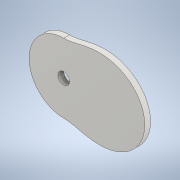
# Autodesk Inventor part: Disc Cam
Saved by Autodesk Inventor 2020.2 (Build 242310000, 310)
## iProperties
Created: 2020-01-12
Part Number: Disc Cam
Material: Stainless Steel, Austenitic
Document SubType Name: Modeling
Designer: robst
Manufacturer: Standard
Standards Organization: Custom
Density: 1 g/cm^3
Appearance: Steel
CustomPartVersion: 1
Author: robst
Autodesk Inventor part; units mm, degrees
ref_plane "YZ Plane" through (0, 0, 0) normal (1, 0, 0) x (0, 1, 0)
ref_plane "XZ Plane" through (0, 0, 0) normal (0, 1, 0) x (-1, 0, 0)
ref_plane "XY Plane" through (0, 0, 0) normal (0, 0, 1) x (1, 0, 0)
sketch "Main Sketch" plane through (0, 0, 0) normal (0, 0, 1) x (1, 0, 0)
  spline S0 degree 5 poles (0, 76.2) (2.4415, 76.2811) (6.8419, 76.4448) (14.3342, 77.0155) (22.5678, 78.9482) (34.573, 81.6506) (46.176, 84.4734) (59.6543, 86.8011) (74.07, 88.0758) (89.5247, 87.6776) (105.5032, 85.1455) (121.5054, 80.094) (136.8136, 72.3306) (150.6942, 61.8554) (162.4064, 48.8865) (171.2981, 33.8414) (176.8529, 17.3087) (178.7423, 0) (176.8529, -17.3087) (171.2981, -33.8414) (162.4064, -48.8865) (150.6941, -61.8554) (136.8137, -72.3305) (121.5052, -80.0941) (105.5037, -85.1453) (89.5236, -87.678) (74.0723, -88.0749) (59.6496, -86.803) (46.1853, -84.4696) (34.1732, -81.5655) (22.4222, -78.8937) (12.4959, -76.6296) (0.313, -76.0937) (-7.0815, -76.2043) (-15.7981, -74.7442) (-23.5043, -72.7115) (-31.1018, -69.794) (-38.1945, -66.1763) (-44.9165, -61.8146) (-51.1259, -56.7839) (-56.7839, -51.1274) (-61.816, -44.9123) (-66.1725, -38.2045) (-69.8032, -31.0785) (-72.6695, -23.6117) (-74.7395, -15.8864) (-75.9906, -7.9869) (-76.4092, 0) (-75.9906, 7.9869) (-74.7395, 15.8864) (-72.6695, 23.6117) (-69.8032, 31.0785) (-66.1725, 38.2045) (-61.8159, 44.9124) (-56.7843, 51.1273) (-51.1251, 56.7841) (-44.9184, 61.8141) (-38.1902, 66.1776) (-31.112, 69.7909) (-23.837, 72.5819) (-16.3649, 74.6032) (-9.6201, 75.7956) (-5.285, 76.037) (-2.0624, 76.1315) (0, 76.2) knots 0 0 0 0 0 0 0.019966 0.033509 0.050708 0.068396 0.086675 0.105572 0.125041 0.144982 0.165276 0.1858 0.206452 0.22715 0.247846 0.26852 0.289177 0.309833 0.330508 0.351204 0.371902 0.392553 0.413078 0.433371 0.453313 0.472781 0.491679 0.509958 0.527646 0.544844 0.561198 0.57685 0.591915 0.606464 0.620518 0.634573 0.648628 0.662683 0.676738 0.690793 0.704848 0.718903 0.732957 0.747012 0.761067 0.775122 0.789177 0.803232 0.817287 0.831342 0.845396 0.859451 0.873506 0.887561 0.901616 0.915671 0.929726 0.943781 0.957835 0.97189 0.983134 1 1 1 1 1 1
  point P0 (22.0134, 78.8258)
  point P1 (33.3701, 81.4116)
  point P2 (45.5354, 84.1258)
  point P3 (58.8273, 86.3979)
  point P4 (73.3136, 87.6269)
  point P5 (88.8039, 87.2207)
  point P6 (104.8783, 84.6627)
  point P7 (120.9362, 79.576)
  point P8 (136.2611, 71.7733)
  point P9 (150.0945, 61.2842)
  point P10 (161.7111, 48.3549)
  point P11 (170.4865, 33.4236)
  point P12 (175.947, 17.0772)
  point P13 (177.8, 0)
  point P14 (175.947, -17.0772)
  point P15 (170.4865, -33.4236)
  point P16 (161.7111, -48.3549)
  point P17 (150.0945, -61.2842)
  point P18 (136.2611, -71.7733)
  point P19 (120.9362, -79.576)
  point P20 (104.8783, -84.6627)
  point P21 (88.8039, -87.2207)
  point P22 (73.3136, -87.6269)
  point P23 (58.8273, -86.3979)
  point P24 (45.5354, -84.1258)
  point P25 (33.3701, -81.4116)
  point P26 (22.0134, -78.8258)
  point P27 (11.002, -76.9174)
  point P28 (0, -76.2)
  point P29 (-7.9651, -75.7826)
  point P30 (-15.8429, -74.5348)
  point P31 (-23.5471, -72.4705)
  point P32 (-30.9933, -69.6122)
  point P33 (-38.1, -65.9911)
  point P34 (-44.7892, -61.6471)
  point P35 (-50.9878, -56.6276)
  point P36 (-56.6276, -50.9878)
  point P37 (-61.6471, -44.7892)
  point P38 (-65.9911, -38.1)
  point P39 (-69.6122, -30.9933)
  point P40 (-72.4705, -23.5471)
  point P41 (-74.5348, -15.8429)
  point P42 (-75.7826, -7.9651)
  point P43 (-76.2, 0)
  point P44 (-75.7826, 7.9651)
  point P45 (-74.5348, 15.8429)
  point P46 (-72.4705, 23.5471)
  point P47 (-69.6122, 30.9933)
  point P48 (-65.9911, 38.1)
  point P49 (-61.6471, 44.7892)
  point P50 (-56.6276, 50.9878)
  point P51 (-50.9878, 56.6276)
  point P52 (-44.7892, 61.6471)
  point P53 (-38.1, 65.9911)
  point P54 (-30.9933, 69.6122)
  point P55 (-23.5471, 72.4705)
  point P56 (-15.8429, 74.5348)
  point P57 (-7.9651, 75.7826)
  constraints: 60 other
extrude "Cam" add sketch "Main Sketch" along normal blind 12.7
sketch "Sketch2" plane through (0, 0, 12.7) normal (0, 0, 1) x (1, 0, 0)
  circle A0 centre (0, 0) radius 12.7
  dimension "d4" = 25.4
  constraints: 1 centre point, 1 coincident
  measures "d4" diameter of A0
extrude "Extrusion2" cut sketch "Sketch2" against normal through all
body "Solid1"
